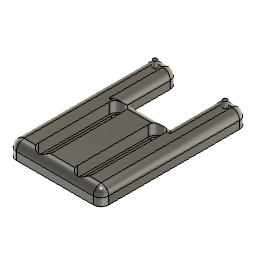
encoder_ext_c3 v2 (Autodesk Fusion 360 design; units mm, degrees)
Autodesk Fusion 360 part; units mm, degrees
note: some values were not read from the file. Set by a fixed rule: which sketch regions a step uses.
sketch "Sketch1" plane through (0, 0, 0) normal (0, 0, 1) x (1, 0, 0)
  line L0 (0, 0) -> (60, 0)
  line L1 (60, 0) -> (60, 95)
  line L2 (60, 95) -> (0, 95)
  line L3 (0, 95) -> (0, 0)
  line L4 (60, 60) -> (0, 60) construction
  line L5 (0, 0) -> (60, 60) construction
  line L6 (0, 60) -> (60, 0) construction
  line L7 (30, 30) -> (30, 60) construction
  line L8 (30, 30) -> (30, 0) construction
  line L9 (42.7, 60) -> (42.7, 0) construction
  line L10 (17.3, 60) -> (17.3, 0) construction
  line L11 (45, 95) -> (45, 60) construction
  line L12 (15, 95) -> (15, 60) construction
  line L13 (52.7, 95) -> (52.7, 60) construction
  line L14 (7.3, 95) -> (7.3, 60) construction
  line L15 (60, 87.783) -> (0, 87.783) construction
  circle A0 centre (52.7, 87.783) radius 1.4
  circle A1 centre (7.3, 87.783) radius 1.4
  line L16 (15, 95) -> (15, 60)
  line L17 (15, 60) -> (45, 60)
  line L18 (45, 60) -> (45, 95)
  line L19 (0, 53) -> (60, 53) construction
  line L20 (0, 7) -> (60, 7) construction
  circle A2 centre (42.7, 53) radius 5
  circle A3 centre (42.7, 7) radius 5
  circle A4 centre (17.3, 7) radius 5
  circle A5 centre (17.3, 53) radius 5
  circle A6 centre (17.3, 53) radius 3.5
  circle A7 centre (17.3, 7) radius 3.5
  circle A8 centre (42.7, 53) radius 3.5
  circle A9 centre (42.7, 7) radius 3.5
  line L21 (12.3, 53) -> (12.3, 7)
  line L22 (22.3, 53) -> (22.3, 7)
  line L23 (13.8, 53) -> (13.8, 7)
  line L24 (20.8, 53) -> (20.8, 7)
  line L25 (37.7, 53) -> (37.7, 7)
  line L26 (39.2, 53) -> (39.2, 7)
  line L27 (46.2, 7) -> (46.2, 53)
  line L28 (47.7, 53) -> (47.7, 7)
  dimension "d1" = 60
  dimension "d2" = 95
  dimension "d3" = 35
  dimension "d4" = 12.7
  dimension "d5" = 12.7
  dimension "d6" = 15
  dimension "d7" = 15
  dimension "d8" = 7.3
  dimension "d9" = 7.3
  dimension "d10" = 27.783
  dimension "d11" = 2.8
  dimension "d12" = 2.8
  dimension "d13" = 7
  dimension "d14" = 7
  dimension "d15" = 10
  dimension "d16" = 10
  dimension "d17" = 10
  dimension "d18" = 10
  dimension "d19" = 7
  dimension "d20" = 7
  dimension "d21" = 7
  dimension "d22" = 7
  constraint horizontal L0
  constraint vertical L1
  constraint horizontal L2
  constraint vertical L3
  constraint coincident L0.start L3.end
  constraint coincident L1 L4.start
  constraint coincident L3 L4.end
  constraint perpendicular L3 L4
  constraint midpoint L5 L7.start
  constraint midpoint L4 L7.end
  constraint midpoint L0 L8.end
  constraint coincident L4 L9.start
  constraint coincident L0 L9.end
  constraint perpendicular L0 L9
  constraint coincident L4 L10.start
  constraint coincident L0 L10.end
  constraint perpendicular L0 L10
  constraint coincident L2 L11.start
  constraint coincident L4 L11.end
  constraint perpendicular L4 L11
  constraint coincident L2 L12.start
  constraint coincident L4 L12.end
  constraint perpendicular L4 L12
  constraint coincident L2 L13.start
  constraint coincident L4 L13.end
  constraint perpendicular L4 L13
  constraint coincident L2 L14.start
  constraint coincident L4 L14.end
  constraint perpendicular L4 L14
  constraint coincident L1 L15.start
  constraint coincident L3 L15.end
  constraint perpendicular L3 L15
  constraint coincident L13 A0.centre
  constraint coincident L15 A0.centre
  constraint coincident L15 A1.centre
  constraint coincident L14 A1.centre
  constraint coincident L3 L19.start
  constraint coincident L1 L19.end
  constraint perpendicular L1 L19
  constraint coincident L3 L20.start
  constraint coincident L1 L20.end
  constraint perpendicular L1 L20
  constraint coincident L9 A2.centre
  constraint coincident L19 A2.centre
  constraint coincident L9 A3.centre
  constraint coincident L20 A3.centre
  constraint coincident L20 A4.centre
  constraint coincident L10 A4.centre
  constraint coincident L19 A5.centre
  constraint coincident L10 A5.centre
  constraint concentric A5 A6
  constraint concentric A4 A7
  constraint concentric A2 A8
  constraint concentric A3 A9
  constraint coincident L19 L21.start
  constraint coincident A5 L21.start
  constraint coincident A4 L21.end
  constraint coincident L20 L21.end
  constraint coincident L19 L22.start
  constraint coincident A5 L22.start
  constraint coincident A4 L22.end
  constraint coincident L20 L22.end
  constraint coincident A6 L23.start
  constraint coincident L19 L23.start
  constraint coincident L20 L23.end
  constraint coincident A7 L23.end
  constraint coincident A6 L24.start
  constraint coincident L19 L24.start
  constraint coincident A7 L24.end
  constraint coincident L20 L24.end
  constraint coincident A2 L25.start
  constraint coincident L19 L25.start
  constraint coincident A3 L25.end
  constraint coincident L20 L25.end
  constraint coincident A8 L26.start
  constraint coincident L19 L26.start
  constraint coincident L20 L26.end
  constraint coincident A9 L26.end
  constraint coincident A9 L27.start
  constraint coincident L20 L27.start
  constraint coincident A8 L27.end
  constraint coincident L19 L27.end
  constraint coincident A2 L28.start
  constraint coincident L19 L28.start
  constraint coincident A3 L28.end
  constraint coincident L20 L28.end
  measures "d1" distance of L0.start L0.end
  measures "d2" distance of L0.start L2.end
  measures "d3" distance of L2 L4
  measures "d4" distance of L7 L9
  measures "d5" distance of L7 L10
  measures "d6" distance of L1 L11
  measures "d7" distance of L3 L12
  measures "d8" distance of L1 L13
  measures "d9" distance of L3 L14
  measures "d10" distance of L4 L15
  measures "d11" diameter of A0
  measures "d12" diameter of A1
  measures "d13" distance of L17 L19
  measures "d14" distance of L0 L20
  measures "d15" diameter of A2
  measures "d16" diameter of A3
  measures "d17" diameter of A4
  measures "d18" diameter of A5
  measures "d19" diameter of A6
  measures "d20" diameter of A7
  measures "d21" diameter of A8
  measures "d22" diameter of A9
extrude "Extrude1" add sketch "Sketch1" along normal blind 10 contours L0 L1 L2 L3 L16 L17 L18 makes body 1
extrude "Extrude2" add sketch "Sketch1" along normal blind 3 contours A2 A8 L26 L27 | A2 A3 L27 L28 | A2 A3 L25 L26 | A3 A9 L26 L27 | A4 A7 L23 L24 | A4 A5 L21 L23 | A4 A5 L22 L24 | A5 A6 L23 L24 picked at (45.1558, 56.7568) picked at (47.1684, 6.5777) picked at (21.7684, 6.5777) picked at (14.3117, 56.3488) bodies 1
extrude "Extrude3" add sketch "Sketch1" along normal blind 14 separate body contours A0 | A1 makes body 2 at (51.8828, 86.6463, 9.3333) makes body 3 at (6.0099, 87.2392, 9.3333)
fillet "Fillet1" radius 5 1 edges at (0, 47.5, 10) on bodies 1
fillet "Fillet2" radius 5 1 edges at (60, 47.5, 10) on bodies 1
fillet "Fillet3" radius 5 5 edges at (0, 0, 2.5) (1.4645, 0, 8.5355) (30, 0, 10) (58.5355, 0, 8.5355) (60, 0, 2.5) on bodies 1
fillet "Fillet4" radius 5 6 edges at (60, 95, 2.5) (58.5355, 95, 8.5355) (50, 95, 10) (10, 95, 10) (1.4645, 95, 8.5355) (0, 95, 2.5) on bodies 1
fillet "Fillet5" radius 5 7 edges at (45, 95, 2.5) (45, 93.5355, 8.5355) (45, 75, 10) (30, 60, 10) (15, 75, 10) (15, 93.5355, 8.5355) (15, 95, 2.5) on bodies 1
